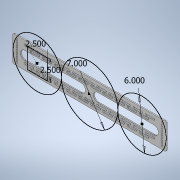
# Autodesk Inventor part: QuickPrototypePlateA
Saved by Autodesk Inventor 2020 (Build 240168000, 168)
## iProperties
Created: 2020-01-06
Part Number: QuickPrototypePlateA
Material: Generic
Document SubType Name: Modeling
Designer: srini
Density: 1 g/cm^3
Appearance: Default
Author: srini
Autodesk Inventor part; units mm, degrees
ref_plane "YZ Plane" through (0, 0, 0) normal (1, 0, 0) x (0, 1, 0)
ref_plane "XZ Plane" through (0, 0, 0) normal (0, 1, 0) x (-1, 0, 0)
ref_plane "XY Plane" through (0, 0, 0) normal (0, 0, 1) x (1, 0, 0)
sketch "Sketch1" plane through (0, 0, 0) normal (0, 0, 1) x (1, 0, 0)
  line L0 (-241.3, 44.45) -> (241.3, 44.45)
  line L1 (241.3, 44.45) -> (241.3, -38.1)
  line L2 (241.3, -38.1) -> (-241.3, -38.1)
  line L3 (-241.3, -38.1) -> (-241.3, 44.45)
  line L4 (-203.2, -19.05) -> (-177.8, -19.05) construction
  line L5 (-203.2, -21.6154) -> (-177.8, -21.6154)
  line L6 (-177.8, -16.4846) -> (-203.2, -16.4846)
  arc A0 (-203.2, -16.4846) -> (-203.2, -21.6154) centre (-203.2, -19.05) ccw
  arc A1 (-177.8, -21.6154) -> (-177.8, -16.4846) centre (-177.8, -19.05) ccw
  line L7 (-203.2, 31.75) -> (-177.8, 31.75) construction
  line L8 (-203.2, 29.1846) -> (-177.8, 29.1846)
  line L9 (-177.8, 34.3154) -> (-203.2, 34.3154)
  arc A2 (-203.2, 34.3154) -> (-203.2, 29.1846) centre (-203.2, 31.75) ccw
  arc A3 (-177.8, 29.1846) -> (-177.8, 34.3154) centre (-177.8, 31.75) ccw
  arc A4 (-139.7, -21.6154) -> (-139.7, -16.4846) centre (-139.7, -19.05) ccw
  arc A5 (-139.7, 29.1846) -> (-139.7, 34.3154) centre (-139.7, 31.75) ccw
  line L10 (-139.7, -16.4846) -> (-165.1, -16.4846)
  line L11 (-165.1, -19.05) -> (-139.7, -19.05) construction
  line L12 (-165.1, -21.6154) -> (-139.7, -21.6154)
  line L13 (-165.1, 29.1846) -> (-139.7, 29.1846)
  line L14 (-165.1, 31.75) -> (-139.7, 31.75) construction
  line L15 (-139.7, 34.3154) -> (-165.1, 34.3154)
  arc A6 (-165.1, -16.4846) -> (-165.1, -21.6154) centre (-165.1, -19.05) ccw
  arc A7 (-165.1, 34.3154) -> (-165.1, 29.1846) centre (-165.1, 31.75) ccw
  arc A8 (-101.6, -21.6154) -> (-101.6, -16.4846) centre (-101.6, -19.05) ccw
  arc A9 (-101.6, 29.1846) -> (-101.6, 34.3154) centre (-101.6, 31.75) ccw
  line L16 (-101.6, -16.4846) -> (-127, -16.4846)
  line L17 (-127, -19.05) -> (-101.6, -19.05) construction
  line L18 (-127, -21.6154) -> (-101.6, -21.6154)
  line L19 (-127, 29.1846) -> (-101.6, 29.1846)
  line L20 (-127, 31.75) -> (-101.6, 31.75) construction
  line L21 (-101.6, 34.3154) -> (-127, 34.3154)
  arc A10 (-127, -16.4846) -> (-127, -21.6154) centre (-127, -19.05) ccw
  arc A11 (-127, 34.3154) -> (-127, 29.1846) centre (-127, 31.75) ccw
  arc A12 (-63.5, -21.6154) -> (-63.5, -16.4846) centre (-63.5, -19.05) ccw
  arc A13 (-63.5, 29.1846) -> (-63.5, 34.3154) centre (-63.5, 31.75) ccw
  line L22 (-63.5, -16.4846) -> (-88.9, -16.4846)
  line L23 (-88.9, -19.05) -> (-63.5, -19.05) construction
  line L24 (-88.9, -21.6154) -> (-63.5, -21.6154)
  line L25 (-88.9, 29.1846) -> (-63.5, 29.1846)
  line L26 (-88.9, 31.75) -> (-63.5, 31.75) construction
  line L27 (-63.5, 34.3154) -> (-88.9, 34.3154)
  arc A14 (-88.9, -16.4846) -> (-88.9, -21.6154) centre (-88.9, -19.05) ccw
  arc A15 (-88.9, 34.3154) -> (-88.9, 29.1846) centre (-88.9, 31.75) ccw
  arc A16 (-25.4, -21.6154) -> (-25.4, -16.4846) centre (-25.4, -19.05) ccw
  arc A17 (-25.4, 29.1846) -> (-25.4, 34.3154) centre (-25.4, 31.75) ccw
  line L28 (-25.4, -16.4846) -> (-50.8, -16.4846)
  line L29 (-50.8, -19.05) -> (-25.4, -19.05) construction
  line L30 (-50.8, -21.6154) -> (-25.4, -21.6154)
  line L31 (-50.8, 29.1846) -> (-25.4, 29.1846)
  line L32 (-50.8, 31.75) -> (-25.4, 31.75) construction
  line L33 (-25.4, 34.3154) -> (-50.8, 34.3154)
  arc A18 (-50.8, -16.4846) -> (-50.8, -21.6154) centre (-50.8, -19.05) ccw
  arc A19 (-50.8, 34.3154) -> (-50.8, 29.1846) centre (-50.8, 31.75) ccw
  arc A20 (12.7, -21.6154) -> (12.7, -16.4846) centre (12.7, -19.05) ccw
  arc A21 (12.7, 29.1846) -> (12.7, 34.3154) centre (12.7, 31.75) ccw
  line L34 (12.7, -16.4846) -> (-12.7, -16.4846)
  line L35 (-12.7, -19.05) -> (12.7, -19.05) construction
  line L36 (-12.7, -21.6154) -> (12.7, -21.6154)
  line L37 (-12.7, 29.1846) -> (12.7, 29.1846)
  line L38 (-12.7, 31.75) -> (12.7, 31.75) construction
  line L39 (12.7, 34.3154) -> (-12.7, 34.3154)
  arc A22 (-12.7, -16.4846) -> (-12.7, -21.6154) centre (-12.7, -19.05) ccw
  arc A23 (-12.7, 34.3154) -> (-12.7, 29.1846) centre (-12.7, 31.75) ccw
  arc A24 (50.8, -21.6154) -> (50.8, -16.4846) centre (50.8, -19.05) ccw
  arc A25 (50.8, 29.1846) -> (50.8, 34.3154) centre (50.8, 31.75) ccw
  line L40 (50.8, -16.4846) -> (25.4, -16.4846)
  line L41 (25.4, -19.05) -> (50.8, -19.05) construction
  line L42 (25.4, -21.6154) -> (50.8, -21.6154)
  line L43 (25.4, 29.1846) -> (50.8, 29.1846)
  line L44 (25.4, 31.75) -> (50.8, 31.75) construction
  line L45 (50.8, 34.3154) -> (25.4, 34.3154)
  arc A26 (25.4, -16.4846) -> (25.4, -21.6154) centre (25.4, -19.05) ccw
  arc A27 (25.4, 34.3154) -> (25.4, 29.1846) centre (25.4, 31.75) ccw
  arc A28 (88.9, -21.6154) -> (88.9, -16.4846) centre (88.9, -19.05) ccw
  arc A29 (88.9, 29.1846) -> (88.9, 34.3154) centre (88.9, 31.75) ccw
  line L46 (88.9, -16.4846) -> (63.5, -16.4846)
  line L47 (63.5, -19.05) -> (88.9, -19.05) construction
  line L48 (63.5, -21.6154) -> (88.9, -21.6154)
  line L49 (63.5, 29.1846) -> (88.9, 29.1846)
  line L50 (63.5, 31.75) -> (88.9, 31.75) construction
  line L51 (88.9, 34.3154) -> (63.5, 34.3154)
  arc A30 (63.5, -16.4846) -> (63.5, -21.6154) centre (63.5, -19.05) ccw
  arc A31 (63.5, 34.3154) -> (63.5, 29.1846) centre (63.5, 31.75) ccw
  arc A32 (127, -21.6154) -> (127, -16.4846) centre (127, -19.05) ccw
  arc A33 (127, 29.1846) -> (127, 34.3154) centre (127, 31.75) ccw
  line L52 (127, -16.4846) -> (101.6, -16.4846)
  line L53 (101.6, -19.05) -> (127, -19.05) construction
  line L54 (101.6, -21.6154) -> (127, -21.6154)
  line L55 (101.6, 29.1846) -> (127, 29.1846)
  line L56 (101.6, 31.75) -> (127, 31.75) construction
  line L57 (127, 34.3154) -> (101.6, 34.3154)
  arc A34 (101.6, -16.4846) -> (101.6, -21.6154) centre (101.6, -19.05) ccw
  arc A35 (101.6, 34.3154) -> (101.6, 29.1846) centre (101.6, 31.75) ccw
  line L58 (-184.15, 24.13) -> (-158.75, 24.13) construction
  line L59 (-184.15, 21.5646) -> (-158.75, 21.5646)
  line L60 (-158.75, 26.6954) -> (-184.15, 26.6954)
  arc A36 (-184.15, 26.6954) -> (-184.15, 21.5646) centre (-184.15, 24.13) ccw
  arc A37 (-158.75, 21.5646) -> (-158.75, 26.6954) centre (-158.75, 24.13) ccw
  line L61 (-184.15, -26.67) -> (-158.75, -26.67) construction
  line L62 (-184.15, -29.2354) -> (-158.75, -29.2354)
  line L63 (-158.75, -24.1046) -> (-184.15, -24.1046)
  arc A38 (-184.15, -24.1046) -> (-184.15, -29.2354) centre (-184.15, -26.67) ccw
  arc A39 (-158.75, -29.2354) -> (-158.75, -24.1046) centre (-158.75, -26.67) ccw
  arc A40 (-146.05, 26.6954) -> (-146.05, 21.5646) centre (-146.05, 24.13) ccw
  line L64 (-120.65, 26.6954) -> (-146.05, 26.6954)
  line L65 (-146.05, 24.13) -> (-120.65, 24.13) construction
  line L66 (-146.05, 21.5646) -> (-120.65, 21.5646)
  arc A41 (-120.65, 21.5646) -> (-120.65, 26.6954) centre (-120.65, 24.13) ccw
  line L67 (-120.65, -24.1046) -> (-146.05, -24.1046)
  line L68 (-146.05, -26.67) -> (-120.65, -26.67) construction
  line L69 (-146.05, -29.2354) -> (-120.65, -29.2354)
  arc A42 (-146.05, -24.1046) -> (-146.05, -29.2354) centre (-146.05, -26.67) ccw
  arc A43 (-120.65, -29.2354) -> (-120.65, -24.1046) centre (-120.65, -26.67) ccw
  arc A44 (-107.95, 26.6954) -> (-107.95, 21.5646) centre (-107.95, 24.13) ccw
  line L70 (-82.55, 26.6954) -> (-107.95, 26.6954)
  line L71 (-107.95, 24.13) -> (-82.55, 24.13) construction
  line L72 (-107.95, 21.5646) -> (-82.55, 21.5646)
  arc A45 (-82.55, 21.5646) -> (-82.55, 26.6954) centre (-82.55, 24.13) ccw
  line L73 (-82.55, -24.1046) -> (-107.95, -24.1046)
  line L74 (-107.95, -26.67) -> (-82.55, -26.67) construction
  line L75 (-107.95, -29.2354) -> (-82.55, -29.2354)
  arc A46 (-107.95, -24.1046) -> (-107.95, -29.2354) centre (-107.95, -26.67) ccw
  arc A47 (-82.55, -29.2354) -> (-82.55, -24.1046) centre (-82.55, -26.67) ccw
  arc A48 (-69.85, 26.6954) -> (-69.85, 21.5646) centre (-69.85, 24.13) ccw
  line L76 (-44.45, 26.6954) -> (-69.85, 26.6954)
  line L77 (-69.85, 24.13) -> (-44.45, 24.13) construction
  line L78 (-69.85, 21.5646) -> (-44.45, 21.5646)
  arc A49 (-44.45, 21.5646) -> (-44.45, 26.6954) centre (-44.45, 24.13) ccw
  line L79 (-44.45, -24.1046) -> (-69.85, -24.1046)
  line L80 (-69.85, -26.67) -> (-44.45, -26.67) construction
  line L81 (-69.85, -29.2354) -> (-44.45, -29.2354)
  arc A50 (-69.85, -24.1046) -> (-69.85, -29.2354) centre (-69.85, -26.67) ccw
  arc A51 (-44.45, -29.2354) -> (-44.45, -24.1046) centre (-44.45, -26.67) ccw
  arc A52 (-31.75, 26.6954) -> (-31.75, 21.5646) centre (-31.75, 24.13) ccw
  line L82 (-6.35, 26.6954) -> (-31.75, 26.6954)
  line L83 (-31.75, 24.13) -> (-6.35, 24.13) construction
  line L84 (-31.75, 21.5646) -> (-6.35, 21.5646)
  arc A53 (-6.35, 21.5646) -> (-6.35, 26.6954) centre (-6.35, 24.13) ccw
  line L85 (-6.35, -24.1046) -> (-31.75, -24.1046)
  line L86 (-31.75, -26.67) -> (-6.35, -26.67) construction
  line L87 (-31.75, -29.2354) -> (-6.35, -29.2354)
  arc A54 (-31.75, -24.1046) -> (-31.75, -29.2354) centre (-31.75, -26.67) ccw
  arc A55 (-6.35, -29.2354) -> (-6.35, -24.1046) centre (-6.35, -26.67) ccw
  arc A56 (6.35, 26.6954) -> (6.35, 21.5646) centre (6.35, 24.13) ccw
  line L88 (31.75, 26.6954) -> (6.35, 26.6954)
  line L89 (6.35, 24.13) -> (31.75, 24.13) construction
  line L90 (6.35, 21.5646) -> (31.75, 21.5646)
  arc A57 (31.75, 21.5646) -> (31.75, 26.6954) centre (31.75, 24.13) ccw
  line L91 (31.75, -24.1046) -> (6.35, -24.1046)
  line L92 (6.35, -26.67) -> (31.75, -26.67) construction
  line L93 (6.35, -29.2354) -> (31.75, -29.2354)
  arc A58 (6.35, -24.1046) -> (6.35, -29.2354) centre (6.35, -26.67) ccw
  arc A59 (31.75, -29.2354) -> (31.75, -24.1046) centre (31.75, -26.67) ccw
  arc A60 (44.45, 26.6954) -> (44.45, 21.5646) centre (44.45, 24.13) ccw
  line L94 (69.85, 26.6954) -> (44.45, 26.6954)
  line L95 (44.45, 24.13) -> (69.85, 24.13) construction
  line L96 (44.45, 21.5646) -> (69.85, 21.5646)
  arc A61 (69.85, 21.5646) -> (69.85, 26.6954) centre (69.85, 24.13) ccw
  line L97 (69.85, -24.1046) -> (44.45, -24.1046)
  line L98 (44.45, -26.67) -> (69.85, -26.67) construction
  line L99 (44.45, -29.2354) -> (69.85, -29.2354)
  arc A62 (44.45, -24.1046) -> (44.45, -29.2354) centre (44.45, -26.67) ccw
  arc A63 (69.85, -29.2354) -> (69.85, -24.1046) centre (69.85, -26.67) ccw
  arc A64 (82.55, 26.6954) -> (82.55, 21.5646) centre (82.55, 24.13) ccw
  line L100 (107.95, 26.6954) -> (82.55, 26.6954)
  line L101 (82.55, 24.13) -> (107.95, 24.13) construction
  line L102 (82.55, 21.5646) -> (107.95, 21.5646)
  arc A65 (107.95, 21.5646) -> (107.95, 26.6954) centre (107.95, 24.13) ccw
  line L103 (107.95, -24.1046) -> (82.55, -24.1046)
  line L104 (82.55, -26.67) -> (107.95, -26.67) construction
  line L105 (82.55, -29.2354) -> (107.95, -29.2354)
  arc A66 (82.55, -24.1046) -> (82.55, -29.2354) centre (82.55, -26.67) ccw
  arc A67 (107.95, -29.2354) -> (107.95, -24.1046) centre (107.95, -26.67) ccw
  arc A68 (120.65, 26.6954) -> (120.65, 21.5646) centre (120.65, 24.13) ccw
  line L106 (146.05, 26.6954) -> (120.65, 26.6954)
  line L107 (120.65, 24.13) -> (146.05, 24.13) construction
  line L108 (120.65, 21.5646) -> (146.05, 21.5646)
  arc A69 (146.05, 21.5646) -> (146.05, 26.6954) centre (146.05, 24.13) ccw
  line L109 (146.05, -24.1046) -> (120.65, -24.1046)
  line L110 (120.65, -26.67) -> (146.05, -26.67) construction
  line L111 (120.65, -29.2354) -> (146.05, -29.2354)
  arc A70 (120.65, -24.1046) -> (120.65, -29.2354) centre (120.65, -26.67) ccw
  arc A71 (146.05, -29.2354) -> (146.05, -24.1046) centre (146.05, -26.67) ccw
  arc A72 (165.1, -21.6154) -> (165.1, -16.4846) centre (165.1, -19.05) ccw
  arc A73 (165.1, 29.1846) -> (165.1, 34.3154) centre (165.1, 31.75) ccw
  line L112 (165.1, -16.4846) -> (139.7, -16.4846)
  line L113 (139.7, -19.05) -> (165.1, -19.05) construction
  line L114 (139.7, -21.6154) -> (165.1, -21.6154)
  line L115 (139.7, 29.1846) -> (165.1, 29.1846)
  line L116 (139.7, 31.75) -> (165.1, 31.75) construction
  line L117 (165.1, 34.3154) -> (139.7, 34.3154)
  arc A74 (139.7, -16.4846) -> (139.7, -21.6154) centre (139.7, -19.05) ccw
  arc A75 (139.7, 34.3154) -> (139.7, 29.1846) centre (139.7, 31.75) ccw
  line L118 (-26.67, 2.54) -> (-203.2, 2.54) construction
  line L119 (-26.67, 16.51) -> (-203.2, 16.51)
  line L120 (-203.2, -11.43) -> (-26.67, -11.43)
  arc A76 (-26.67, -11.43) -> (-26.67, 16.51) centre (-26.67, 2.54) ccw
  arc A77 (-203.2, 16.51) -> (-203.2, -11.43) centre (-203.2, 2.54) ccw
  line L121 (0, 44.45) -> (0, -38.1) construction
  line L122 (26.67, 2.54) -> (203.2, 2.54) construction
  line L123 (26.67, 16.51) -> (203.2, 16.51)
  line L124 (203.2, -11.43) -> (26.67, -11.43)
  arc A78 (26.67, 16.51) -> (26.67, -11.43) centre (26.67, 2.54) ccw
  arc A79 (203.2, -11.43) -> (203.2, 16.51) centre (203.2, 2.54) ccw
  arc A80 (203.2, -21.6154) -> (203.2, -16.4846) centre (203.2, -19.05) ccw
  arc A81 (203.2, 29.1846) -> (203.2, 34.3154) centre (203.2, 31.75) ccw
  line L125 (203.2, -16.4846) -> (177.8, -16.4846)
  line L126 (177.8, -19.05) -> (203.2, -19.05) construction
  line L127 (177.8, -21.6154) -> (203.2, -21.6154)
  line L128 (177.8, 29.1846) -> (203.2, 29.1846)
  line L129 (177.8, 31.75) -> (203.2, 31.75) construction
  line L130 (203.2, 34.3154) -> (177.8, 34.3154)
  arc A82 (177.8, -16.4846) -> (177.8, -21.6154) centre (177.8, -19.05) ccw
  arc A83 (177.8, 34.3154) -> (177.8, 29.1846) centre (177.8, 31.75) ccw
  arc A84 (158.75, 26.6954) -> (158.75, 21.5646) centre (158.75, 24.13) ccw
  line L131 (184.15, 26.6954) -> (158.75, 26.6954)
  line L132 (158.75, 24.13) -> (184.15, 24.13) construction
  line L133 (158.75, 21.5646) -> (184.15, 21.5646)
  arc A85 (184.15, 21.5646) -> (184.15, 26.6954) centre (184.15, 24.13) ccw
  line L134 (184.15, -24.1046) -> (158.75, -24.1046)
  line L135 (158.75, -26.67) -> (184.15, -26.67) construction
  line L136 (158.75, -29.2354) -> (184.15, -29.2354)
  arc A86 (158.75, -24.1046) -> (158.75, -29.2354) centre (158.75, -26.67) ccw
  arc A87 (184.15, -29.2354) -> (184.15, -24.1046) centre (184.15, -26.67) ccw
  circle A88 centre (-228.6, 34.925) radius 2.5527
  circle A89 centre (-228.6, 28.575) radius 2.5527
  circle A90 centre (-228.6, 22.225) radius 2.5527
  circle A91 centre (-228.6, 15.875) radius 2.5527
  circle A92 centre (-228.6, 9.525) radius 2.5527
  circle A93 centre (-228.6, 3.175) radius 2.5527
  circle A94 centre (228.6, 34.925) radius 2.5527
  circle A95 centre (228.6, 28.575) radius 2.5527
  circle A96 centre (228.6, 22.225) radius 2.5527
  circle A97 centre (228.6, 15.875) radius 2.5527
  circle A98 centre (228.6, 9.525) radius 2.5527
  circle A99 centre (228.6, 3.175) radius 2.5527
  circle A100 centre (-228.6, -3.175) radius 2.5527
  circle A101 centre (228.6, -3.175) radius 2.5527
  circle A102 centre (-228.6, -9.525) radius 2.5527
  circle A103 centre (228.6, -9.525) radius 2.5527
  circle A104 centre (-228.6, -15.875) radius 2.5527
  circle A105 centre (228.6, -15.875) radius 2.5527
  circle A106 centre (-228.6, -22.225) radius 2.5527
  circle A107 centre (228.6, -22.225) radius 2.5527
  circle A108 centre (-228.6, -28.575) radius 2.5527
  circle A109 centre (228.6, -28.575) radius 2.5527
  point P0 (0, 0)
  point P1 (-190.5, -19.05)
  point P2 (-190.5, 31.75)
  point P3 (-152.4, -19.05)
  point P4 (-152.4, 31.75)
  point P5 (-114.3, -19.05)
  point P6 (-114.3, 31.75)
  point P7 (-76.2, -19.05)
  point P8 (-76.2, 31.75)
  point P9 (-38.1, -19.05)
  point P10 (-38.1, 31.75)
  point P11 (0, -19.05)
  point P12 (0, 31.75)
  point P13 (38.1, -19.05)
  point P14 (38.1, 31.75)
  point P15 (76.2, -19.05)
  point P16 (76.2, 31.75)
  point P17 (114.3, -19.05)
  point P18 (114.3, 31.75)
  point P19 (-171.45, 24.13)
  point P20 (-171.45, -26.67)
  point P21 (-133.35, 24.13)
  point P22 (-133.35, -26.67)
  point P23 (-95.25, 24.13)
  point P24 (-95.25, -26.67)
  point P25 (-57.15, 24.13)
  point P26 (-57.15, -26.67)
  point P27 (-19.05, 24.13)
  point P28 (-19.05, -26.67)
  point P29 (19.05, 24.13)
  point P30 (19.05, -26.67)
  point P31 (57.15, 24.13)
  point P32 (57.15, -26.67)
  point P33 (95.25, 24.13)
  point P34 (95.25, -26.67)
  point P35 (133.35, 24.13)
  point P36 (133.35, -26.67)
  point P37 (152.4, -19.05)
  point P38 (152.4, 31.75)
  point P39 (-114.935, 2.54)
  point P40 (114.935, 2.54)
  point P41 (190.5, -19.05)
  point P42 (190.5, 31.75)
  point P43 (171.45, 24.13)
  point P44 (171.45, -26.67)
  dimension "d0" = 482.6
  dimension "d1" = 82.55
  dimension "d2" = 241.3
  dimension "d3" = 44.45
  dimension "d4" = 2.5654
  dimension "d5" = 25.4
  dimension "d6" = 50.8
  dimension "d7" = 38.1
  dimension "d8" = 31.75
  dimension "d11" = 38.1
  dimension "d16" = 19.05
  dimension "d17" = 50.8
  dimension "d18" = 7.62
  dimension "d19" = 24.13
  dimension "d22" = 38.1
  dimension "d34" = 13.97
  dimension "d35" = 29.21
  dimension "d38" = 26.67
  dimension "d62" = 12.7
  dimension "d63" = 5.1054
  dimension "d64" = 9.525
  dimension "d67" = 6.35
  dimension "d70" = 457.2
  constraints: 362 end point, 176 point on circle, 110 centre point, 20 tangent, 12 parallel, 7 horizontal, 7 midpoint, 7 symmetric about line, 3 equal radius, 3 vertical alignment, 1 perpendicular, 1 vertical, 500 other
  measures "d0" distance of L0.start L0.end
  measures "d1" distance of L2.end L0.start
  measures "d2" distance from line of L3 point (0, 0)
  measures "d3" distance from line of point (0, 0) L0
  measures "d4" radius of A3
  measures "d5" distance of L7.start L7.end
  measures "d6" distance between parallel lines of L4 L7
  measures "d7" distance from line of L7.start L3
  measures "d8" distance from line of L7 point (0, 0)
  measures "d11" distance of L6.start L10.start
  measures "d16" horizontal distance of L58.start L7.start
  measures "d17" distance between parallel lines of L61 L58
  measures "d18" distance between parallel lines of L58 L7
  measures "d19" distance from line of L58 point (0, 0)
  measures "d22" distance of L60.end L64.end
  measures "d34" radius of A76
  measures "d35" distance between parallel lines of L118 L7
  measures "d38" horizontal distance of L118.start point (0, 0)
  measures "d62" distance from line of A88.centre L3
  measures "d63" diameter of A88
  measures "d64" distance from line of A88.centre L0
  measures "d67" distance of A88.centre A89.centre
  measures "d70" distance of A88.centre A94.centre
extrude "Extrusion1" add sketch "Sketch1" along normal blind 3.175
sketch "Sketch2" plane through (0, 0, 3.175) normal (0, 0, 1) x (1, 0, 0)
  circle A0 centre (0, 0) radius 88.9
  circle A1 centre (-165.1, 0) radius 76.2
  circle A2 centre (165.1, 0) radius 76.2
  line L0 (-196.85, 31.75) -> (-133.35, 31.75)
  line L1 (-133.35, 31.75) -> (-133.35, -31.75)
  line L2 (-133.35, -31.75) -> (-196.85, -31.75)
  line L3 (-196.85, -31.75) -> (-196.85, 31.75)
  line L4 (-196.85, 31.75) -> (-133.35, -31.75) construction
  line L5 (-133.35, 31.75) -> (-196.85, -31.75) construction
  dimension "d49" = 177.8
  dimension "d51" = 152.4
  dimension "d53" = 63.5
  dimension "d54" = 63.5
  constraints: 12 end point, 3 centre point, 2 horizontal alignment, 2 midpoint, 2 parallel, 2 tangent, 1 coincident, 1 equal radius, 1 horizontal, 1 perpendicular
  measures "d49" diameter of A0
  measures "d51" diameter of A2
  measures "d53" distance of L0.start L0.end
  measures "d54" distance of L0.end L1.end
fillet "Fillet1" radius 3.175 4 edges at (241.3, -38.1, 1.5875) (241.3, 44.45, 1.5875) (-241.3, 44.45, 1.5875) (-241.3, -38.1, 1.5875)
equation "\"d2\" = 0.5 * d0"
body "Solid1"
